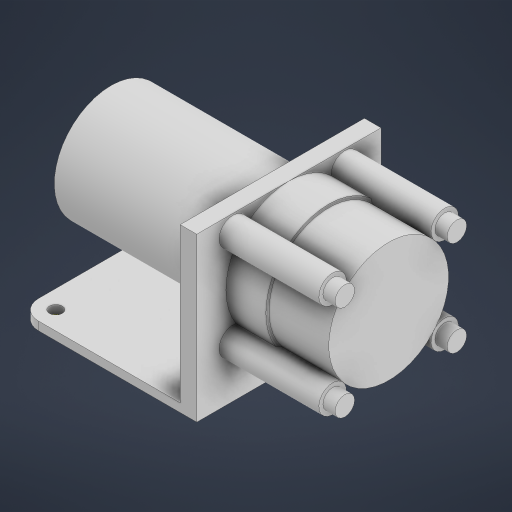
# Autodesk Inventor part: Pump
Saved by Autodesk Inventor 2024.3 (Build 283343000, 343)
## iProperties
Created: 2024-06-12
Part Number: Pump
Material: Generic
Document SubType Name: Modeling
Designer: braed
Density: 1 g/cm^3
Appearance: Default
Author: braed
Autodesk Inventor part; units mm, degrees
ref_plane "YZ Plane" through (0, 0, 0) normal (1, 0, 0) x (0, 1, 0)
ref_plane "XZ Plane" through (0, 0, 0) normal (0, 1, 0) x (-1, 0, 0)
ref_plane "XY Plane" through (0, 0, 0) normal (0, 0, 1) x (1, 0, 0)
sketch "Sketch1" plane through (0, 0, 0) normal (1, 0, 0) x (0, 1, 0)
  circle A0 centre (0, 0) radius 18.5
  dimension "d0" = 37
  constraints: 1 centre point, 1 coincident
  measures "d0" diameter of A0
extrude "Extrusion1" add sketch "Sketch1" along normal blind 52.5
sketch "Sketch2" plane through (52.5, 0, 0) normal (1, 0, 0) x (0, 0, -1)
  circle A0 centre (0, 0) radius 18.5 projected
  line L0 (0, 18.5) -> (0, 15.5) construction
  line L1 (0, 15.5) -> (18.25, 15.5) construction
  line L2 (0, 15.5) -> (-18.25, 15.5) construction
  circle A1 centre (18.25, 15.5) radius 2.1
  circle A2 centre (-18.25, 15.5) radius 2.1
  line L3 (0, 15.5) -> (0, 20.5) construction
  line L4 (0, 20.5) -> (30, 20.5) construction
  line L5 (0, 20.5) -> (-30, 20.5) construction
  line L6 (-30, 20.5) -> (30, 20.5)
  line L7 (30, 20.5) -> (30, -32.5)
  line L8 (30, -32.5) -> (-30, -32.5)
  line L9 (-30, -32.5) -> (-30, 20.5)
  dimension "d3" = 3
  dimension "d4" = 18.25
  dimension "d5" = 4.2
  dimension "d6" = 5
  dimension "d7" = 30
  dimension "d8" = 53
  constraints: 20 end point, 3 symmetric about line, 2 centre point, 2 horizontal, 2 parallel, 2 perpendicular, 2 vertical, 1 coincident, 1 vertical alignment, 2 other
  measures "d3" distance of L0.start L0.end
  measures "d4" distance of L0.end L1.end
  measures "d5" diameter of A1
  measures "d6" distance of L0.end L3.end
  measures "d7" distance of L3.end L4.end
  measures "d8" distance of L6.end L7.end
extrude "Extrusion2" add sketch "Sketch2" along normal blind 5.4 contours A0 | L6 L7 L8 L9
sketch "Sketch3" plane through (52.5, 0, 0) normal (-1, 0, 0) x (0, 0, 1)
  line L0 (30, 20.5) -> (30, -32.5) projected
  line L1 (-30, -32.5) -> (-30, 20.5) projected
  line L2 (30, -32.5) -> (-30, -32.5)
  line L3 (-30, -32.5) -> (-30, -29.75)
  line L4 (-30, -29.75) -> (30, -29.75)
  line L5 (30, -29.75) -> (30, -32.5)
  point P0 (0, 0)
  dimension "d11" = 2.75
  constraints: 8 end point, 2 parallel, 1 horizontal, 1 perpendicular, 1 point on line
  measures "d11" distance of L2.end L3.end
extrude "Extrusion3" add sketch "Sketch3" along normal blind 52.5
sketch "Sketch4" plane through (57.9, 0, 0) normal (1, 0, 0) x (0, 0, -1)
  circle A0 centre (-18.25, 15.5) radius 2.1 projected
  circle A1 centre (18.25, 15.5) radius 2.1 projected
  circle A2 centre (0, 0) radius 18.5 construction
  line L0 (0, 0) -> (11.8041, 0) construction
  circle A3 centre (-18.25, -15.5) radius 2.1
  circle A4 centre (18.25, -15.5) radius 2.1
  constraints: 2 centre point, 2 end point, 2 symmetric about line, 1 horizontal, 2 other
extrude "Extrusion4" cut sketch "Sketch4" against normal through all contours A3 | A4
sketch "Sketch5" plane through (52.5, -29.75, 30) normal (0, 1, 0) x (1, 0, 0)
  line L0 (-52.5, 0) -> (-52.5, 60) construction
  line L1 (-52.5, 0) -> (-46.5, 0) construction
  line L2 (0, 0) -> (-52.5, 0) construction
  line L3 (-46.5, 0) -> (-46.5, 6) construction
  circle A0 centre (-46.5, 6) radius 2.1
  line L4 (-52.5, 30) -> (-49.5, 30) construction
  line L5 (-52.5, 30) -> (-49.5, 30) construction
  circle A1 centre (-46.5, 54) radius 2.1
  dimension "d16" = 6
  dimension "d17" = 6
  dimension "d18" = 4.2
  dimension "d19" = 0
  constraints: 8 end point, 2 centre point, 1 coincident, 1 collinear, 1 horizontal, 1 perpendicular, 1 point on line, 1 symmetric about line, 1 other
  measures "d16" distance of L0.start L1.end
  measures "d17" distance of L1.end L3.end
  measures "d18" diameter of A0
  measures "d19" distance between parallel lines of L4 L5
extrude "Extrusion5" cut sketch "Sketch5" against normal through all
fillet "Fillet1" radius 6.35 2 edges at (0, -31.125, 30) (0, -31.125, -30)
sketch "Sketch6" plane through (57.9, 0, 0) normal (1, 0, 0) x (0, 0, -1)
  circle A0 centre (-18.25, 15.5) radius 2.1 projected
  circle A1 centre (18.25, 15.5) radius 2.1 projected
  circle A2 centre (18.25, -15.5) radius 2.1 projected
  circle A3 centre (-18.25, -15.5) radius 2.1 projected
  line L0 (-18.25, 15.5) -> (18.25, -15.5) construction
  circle A4 centre (0, 0) radius 19.5
  circle A5 centre (-18.25, 15.5) radius 4.5
  circle A6 centre (18.25, 15.5) radius 4.5
  circle A7 centre (18.25, -15.5) radius 4.5
  circle A8 centre (-18.25, -15.5) radius 4.5
  point P0 (-15.2684, -12.1295)
  point P1 (-14.4413, -13.1034)
  point P2 (14.4413, -13.1034)
  point P3 (15.2684, -12.1295)
  point P4 (15.2684, 12.1295)
  point P5 (14.4413, 13.1034)
  point P6 (-14.4413, 13.1034)
  point P7 (-15.2684, 12.1295)
  dimension "d23" = 39
  dimension "d24" = 9
  dimension "d25" = 9
  dimension "d26" = 9
  dimension "d27" = 9
  constraints: 5 centre point, 5 coincident, 2 end point
  measures "d23" diameter of A4
  measures "d24" diameter of A5
  measures "d25" diameter of A6
  measures "d26" diameter of A7
  measures "d27" diameter of A8
extrude "Extrusion6" add sketch "Sketch6" along normal blind 32.5 contours A4 A7 A8 A5 A6 | A4 A6 | A7 A4 | A4 A5 | A8 A4 picked at (21.8842, 16.0341) picked at (21.8842, -16.0341) picked at (-14.6159, 16.0344) picked at (-14.6159, -16.0344)
sketch "Sketch7" plane through (57.9, 0, 0) normal (1, 0, 0) x (0, 0, -1)
  circle A0 centre (0, 0) radius 18.5 projected
  circle A1 centre (0, 0) radius 20.5
  constraints: 1 centre point, 1 coincident
extrude "Extrusion7" add sketch "Sketch7" along normal blind 13
sketch "Sketch8" plane through (90.4, 0, 0) normal (1, 0, 0) x (0, 0, -1)
  circle A0 centre (-18.25, 15.5) radius 2.1 projected
  circle A1 centre (-18.25, 15.5) radius 3.175
  circle A2 centre (18.25, 15.5) radius 2.1 projected
  circle A3 centre (18.25, 15.5) radius 3.175
  line L0 (0, 0) -> (9.867, 0) construction
  circle A4 centre (-18.25, -15.5) radius 3.175
  circle A5 centre (18.25, -15.5) radius 3.175
  dimension "d32" = 6.35
  dimension "d33" = 6.35
  constraints: 4 centre point, 2 coincident, 2 end point, 2 symmetric about line, 1 horizontal, 2 other
  measures "d32" diameter of A1
  measures "d33" diameter of A3
extrude "Extrusion8" add sketch "Sketch8" along normal blind 3.9688 contours A0 | A1 | A2 | A3 | A4 | A5
sketch "Sketch9" plane through (57.9, -32.5, -30) normal (0, -1, 0) x (1, 0, 0)
  circle A0 centre (-51.9, 6) radius 2.1 construction
  circle A1 centre (-51.9, 54) radius 2.1 construction
  line L0 (-51.9, 6) -> (-51.9, 54) construction
  point P0 (-57.9, 30)
  constraints: 2 end point, 1 vertical
body "Solid1"
